Autodesk Fusion 360 part; units mm, degrees
(part 2 of 2)
  arc A190 (-205, -267.5) -> (-205, -272.5) centre (-205, -270) ccw
  line L195 (-205, -267.5) -> (-195, -267.5)
  arc A191 (-195, -272.5) -> (-195, -267.5) centre (-195, -270) ccw
  line L196 (-155, -272.5) -> (-165, -272.5)
  arc A192 (-165, -267.5) -> (-165, -272.5) centre (-165, -270) ccw
  line L197 (-165, -267.5) -> (-155, -267.5)
  arc A193 (-155, -272.5) -> (-155, -267.5) centre (-155, -270) ccw
  line L198 (-195, -312.5) -> (-205, -312.5)
  arc A194 (-205, -307.5) -> (-205, -312.5) centre (-205, -310) ccw
  line L199 (-205, -307.5) -> (-195, -307.5)
  arc A195 (-195, -312.5) -> (-195, -307.5) centre (-195, -310) ccw
  arc A196 (-255, -172.5) -> (-255, -167.5) centre (-255, -170) ccw
  line L200 (-255, -172.5) -> (-265, -172.5)
  arc A197 (-265, -167.5) -> (-265, -172.5) centre (-265, -170) ccw
  line L201 (-265, -167.5) -> (-255, -167.5)
  line L202 (-35, -312.5) -> (-45, -312.5)
  arc A198 (-45, -307.5) -> (-45, -312.5) centre (-45, -310) ccw
  line L203 (-45, -307.5) -> (-35, -307.5)
  arc A199 (-35, -312.5) -> (-35, -307.5) centre (-35, -310) ccw
  arc A200 (-215, -52.5) -> (-215, -47.5) centre (-215, -50) ccw
  line L204 (-215, -52.5) -> (-225, -52.5)
  arc A201 (-225, -47.5) -> (-225, -52.5) centre (-225, -50) ccw
  line L205 (-225, -47.5) -> (-215, -47.5)
  arc A202 (-55, -252.5) -> (-55, -247.5) centre (-55, -250) ccw
  line L206 (-55, -252.5) -> (-65, -252.5)
  arc A203 (-65, -247.5) -> (-65, -252.5) centre (-65, -250) ccw
  line L207 (-65, -247.5) -> (-55, -247.5)
  arc A204 (-175, -92.5) -> (-175, -87.5) centre (-175, -90) ccw
  line L208 (-175, -92.5) -> (-185, -92.5)
  arc A205 (-185, -87.5) -> (-185, -92.5) centre (-185, -90) ccw
  line L209 (-185, -87.5) -> (-175, -87.5)
  arc A206 (-55, -132.5) -> (-55, -127.5) centre (-55, -130) ccw
  line L210 (-55, -132.5) -> (-65, -132.5)
  arc A207 (-65, -127.5) -> (-65, -132.5) centre (-65, -130) ccw
  line L211 (-65, -127.5) -> (-55, -127.5)
  arc A208 (-95, -292.5) -> (-95, -287.5) centre (-95, -290) ccw
  line L212 (-95, -292.5) -> (-105, -292.5)
  arc A209 (-105, -287.5) -> (-105, -292.5) centre (-105, -290) ccw
  line L213 (-105, -287.5) -> (-95, -287.5)
  arc A210 (-255, -12.5) -> (-255, -7.5) centre (-255, -10) ccw
  line L214 (-255, -12.5) -> (-265, -12.5)
  arc A211 (-265, -7.5) -> (-265, -12.5) centre (-265, -10) ccw
  line L215 (-265, -7.5) -> (-255, -7.5)
  circle A212 centre (-165, -145) radius 4.5
  circle A213 centre (-90, -120) radius 4.5
  circle A214 centre (-165, -195) radius 4.5
  circle A215 centre (-190, -120) radius 4.5
  circle A216 centre (-115, -145) radius 4.5
  circle A217 centre (-190, -220) radius 4.5
  circle A218 centre (-90, -220) radius 4.5
  circle A219 centre (-115, -195) radius 4.5
  arc A220 (0, -8) -> (-8, 0) centre (-8, -8) ccw
  line L216 (-8, 0) -> (-272, 0)
  arc A221 (-272, 0) -> (-280, -8) centre (-272, -8) ccw
  line L217 (-280, -8) -> (-280, -332)
  arc A222 (-280, -332) -> (-272, -340) centre (-272, -332) ccw
  line L218 (-272, -340) -> (-8, -340)
  arc A223 (-8, -340) -> (0, -332) centre (-8, -332) ccw
  line L219 (0, -332) -> (0, -8)
equation "hole_size = 9 mm"
equation "d10 = hole_size"
named bodies: "SkadisVesaHolder"
